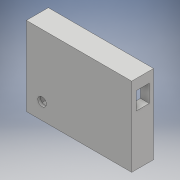
# Autodesk Inventor part: Case_Bottom_Part
Saved by Autodesk Inventor 2017 (Build 210142000, 142)
## iProperties
Created: 2020-01-23
Part Number: Case_Bottom_Part
Material: Generic
Document SubType Name: Modeling
Designer: Manny
Density: 1 g/cm^3
Appearance: Default
Author: Manny
Autodesk Inventor part; units mm, degrees
ref_plane "YZ Plane" through (0, 0, 0) normal (1, 0, 0) x (0, 1, 0)
ref_plane "XZ Plane" through (0, 0, 0) normal (0, 1, 0) x (-1, 0, 0)
ref_plane "XY Plane" through (0, 0, 0) normal (0, 0, 1) x (1, 0, 0)
sketch "Sketch1" plane through (0, 0, 0) normal (0, 1, 0) x (-1, 0, 0)
  line L0 (120, 43.6082) -> (0, 43.6082)
  line L1 (0, 43.6082) -> (0, -46.3918)
  line L2 (0, -46.3918) -> (120, -46.3918)
  line L3 (120, -46.3918) -> (120, 43.6082)
  point P0 (0, 0)
  dimension "d0" = 90
  dimension "d1" = 120
  dimension "d2" = 0
  constraints: 8 end point, 2 parallel, 1 horizontal, 1 perpendicular
  measures "d0" distance of L2.end L0.start
  measures "d1" distance of L1.end L2.end
  measures "d2" distance from line of point (0, 0) L1
extrude "Extrusion1" add sketch "Sketch1" along normal blind 25
sketch "Sketch2" plane through (0, 25, 0) normal (0, 1, 0) x (1, 0, 0)
  line L0 (-110, -33.6082) -> (-10, -33.6082)
  line L1 (-10, -33.6082) -> (-10, 36.3918)
  line L2 (-10, 36.3918) -> (-110, 36.3918)
  line L3 (-110, 36.3918) -> (-110, -33.6082)
  line L4 (-120, -43.6082) -> (0, -43.6082) projected
  line L5 (0, 46.3918) -> (-120, 46.3918) projected
  line L6 (-120, 46.3918) -> (-120, -43.6082) projected
  line L7 (0, -43.6082) -> (0, 46.3918) projected
  point P0 (0, 0)
  dimension "d5" = 10
  dimension "d6" = 10
  dimension "d7" = 10
  dimension "d8" = 10
  constraints: 8 end point, 2 parallel, 1 horizontal, 1 perpendicular
  measures "d5" distance between parallel lines of L0 L4
  measures "d6" distance between parallel lines of L5 L2
  measures "d7" distance between parallel lines of L6 L3
  measures "d8" distance between parallel lines of L7 L1
extrude "Extrusion2" cut sketch "Sketch2" against normal blind 22 contours L3 L2 L1 L0
sketch "Sketch4" plane through (0, 0, 43.6082) normal (1, 0, 0) x (0, 0, -1)
  line L0 (12, 20) -> (32, 20)
  line L1 (32, 20) -> (32, 5)
  line L2 (32, 5) -> (12, 5)
  line L3 (12, 5) -> (12, 20)
  line L4 (0, 25) -> (90, 25) projected
  line L5 (0, 0) -> (90, 0) projected
  line L6 (90, 0) -> (90, 25) projected
  line L7 (0, 0) -> (0, 25) projected
  point P0 (43.6082, 0)
  dimension "d13" = 5
  dimension "d14" = 5
  dimension "d16" = 20
  dimension "d19" = 12
  constraints: 8 end point, 2 parallel, 1 horizontal, 1 perpendicular
  measures "d13" distance between parallel lines of L4 L0
  measures "d14" distance between parallel lines of L5 L2
  measures "d16" distance of L0.start L0.end
  measures "d19" distance between parallel lines of L7 L3
extrude "Extrusion3" cut sketch "Sketch4" against normal blind 22 contours L0 L1 L2 L3
sketch "Sketch5" plane through (0, 3, 0) normal (0, 1, 0) x (1, 0, 0)
  circle A0 centre (-102.0989, 27.7281) radius 4.8843
  line L0 (-110, -33.6082) -> (-110, 36.3918) projected
  line L1 (-110, 36.3918) -> (-10, 36.3918) projected
  point P0 (0, 0)
  dimension "d20" = 7.9011
  dimension "d21" = 8.6636
  constraints: 1 centre point
  measures "d20" distance from line of L0 A0.centre
  measures "d21" distance from line of L1 A0.centre
extrude "Extrusion4" cut sketch "Sketch5" against normal blind 22
body "Solid1"
